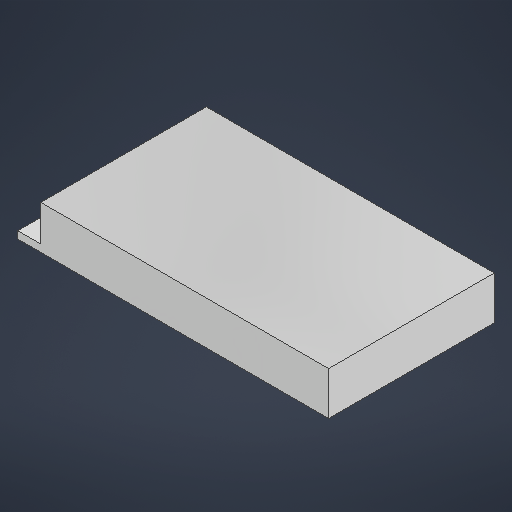
# Autodesk Inventor part: Stepper Power Supply
Saved by Autodesk Inventor 2025.1 (Build 291241000, 241)
## iProperties
Created: 2025-02-09
Part Number: Stepper Power Supply
Material: Generic
Document SubType Name: Modeling
Designer: jerem
Density: 1 g/cm^3
Appearance: Default
Author: jerem
Autodesk Inventor part; units mm, degrees
ref_plane "YZ Plane" through (0, 0, 0) normal (1, 0, 0) x (0, 1, 0)
ref_plane "XZ Plane" through (0, 0, 0) normal (0, 1, 0) x (-1, 0, 0)
ref_plane "XY Plane" through (0, 0, 0) normal (0, 0, 1) x (1, 0, 0)
sketch "Sketch1" plane through (0, 0, 0) normal (0, 1, 0) x (-1, 0, 0)
  line L0 (-107.95, 57.5) -> (107.95, 57.5)
  line L1 (107.95, 57.5) -> (107.95, -57.5)
  line L2 (107.95, -57.5) -> (-107.95, -57.5)
  line L3 (-107.95, -57.5) -> (-107.95, 57.5)
  line L4 (-107.95, 57.5) -> (107.95, -57.5) construction
  line L5 (107.95, 57.5) -> (-107.95, -57.5) construction
  point P0 (0, 0)
  dimension "d0" = 215.9
  dimension "d1" = 115
  constraints: 12 end point, 2 midpoint, 2 parallel, 1 horizontal, 1 perpendicular
  measures "d0" distance of L1.end L2.end
  measures "d1" distance of L0.end L1.end
extrude "Extrusion1" add sketch "Sketch1" along normal blind 30
sketch "Sketch2" plane through (0, 30, 0) normal (0, 1, 0) x (1, 0, 0)
  line L0 (107.95, 57.5) -> (-107.95, 57.5) projected
  line L1 (-107.95, 57.5) -> (-107.95, -57.5) projected
  line L2 (-107.95, -57.5) -> (107.95, -57.5) projected
  line L3 (107.95, -57.5) -> (107.95, 57.5) projected
  line L4 (-91.95, 57.5) -> (-91.95, -57.5)
  point P0 (0, 0)
  dimension "d4" = 16
  constraints: 2 end point, 2 point on line, 1 perpendicular
  measures "d4" distance between parallel lines of L1 L4
extrude "Extrusion2" cut sketch "Sketch2" against normal blind 25 contours L4 L2 L1 L0
sketch "Sketch3" plane through (0, 0, 0) normal (0, -1, 0) x (1, 0, 0)
  line L0 (-74.05, 25) -> (75.95, 25) construction
  line L1 (75.95, 25) -> (75.95, -25) construction
  line L2 (107.95, 57.5) -> (107.95, -57.5) construction
  line L3 (0, 0) -> (75.95, 0) construction
  circle A0 centre (-74.05, 25) radius 2
  circle A1 centre (75.95, 25) radius 2
  circle A2 centre (75.95, -25) radius 2
  line L4 (-74.05, 25) -> (-74.05, -25) construction
  circle A3 centre (-74.05, -25) radius 2
  line L5 (107.95, -57.5) -> (-107.95, -57.5) construction
  line L6 (107.95, 57.5) -> (107.95, -57.5) projected
  line L7 (-107.95, 57.5) -> (107.95, 57.5) construction
  line L8 (-107.95, -57.5) -> (-107.95, 57.5) construction
  dimension "d7" = 150
  dimension "d8" = 50
  dimension "d9" = 32
  dimension "d10" = 4
  constraints: 8 end point, 4 centre point, 4 coincident, 3 equal radius, 2 vertical, 1 horizontal, 1 midpoint, 1 parallel, 1 perpendicular
  measures "d7" distance of L0.start L0.end
  measures "d8" distance of L0.end L1.end
  measures "d9" distance between parallel lines of L2 L1
  measures "d10" diameter of A0
extrude "Extrusion3" cut sketch "Sketch3" against normal blind 4
body "Solid1"
